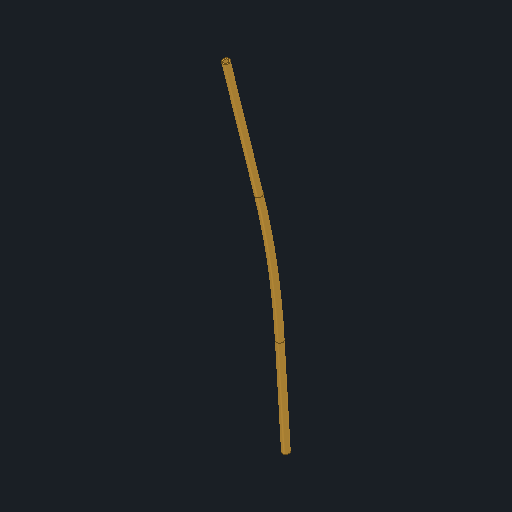
# Autodesk Inventor part: prop_shaft
Saved by Autodesk Inventor 2023 (Build 270158030, 158C)
## iProperties
Created: 2022-04-18
Part Number: prop_shaft
Material: Generic
Document SubType Name: Modeling
Designer: kardo
Density: 1 g/cm^3
Appearance: Brass - Prop shaft
Author: kardo
Autodesk Inventor part; units mm, degrees
ref_plane "YZ Plane" through (0, 0, 0) normal (1, 0, 0) x (0, 1, 0)
ref_plane "XZ Plane" through (0, 0, 0) normal (0, 1, 0) x (-1, 0, 0)
ref_plane "XY Plane" through (0, 0, 0) normal (0, 0, 1) x (1, 0, 0)
derived "stencil_frame.ipt"
sketch "sk_drivetrain_profile" plane through (6, 0, 0) normal (1, 0, 0) x (0, 1, 0)
  line L0 (-547.3485, 0) -> (393.091, 0) construction
  line L1 (-363, 4666.1952) -> (-363, -2045.0469) construction
  line L2 (0, 4666.1952) -> (0, -2045.0469) construction
  line L3 (-140.6277, 54.4571) -> (-133.8539, 27.2888)
  line L4 (-388, 0) -> (-343.0839, 2.7472)
  line L5 (-137.2408, 40.8729) -> (-226.9463, 18.5069)
  line L6 (-320.2745, 4.1423) -> (-272.9504, 7.0367) construction
  line L7 (-272.9504, 7.0367) -> (-226.9463, 18.5069) construction
  line L8 (-133.8539, 27.2888) -> (-133.8539, 22.2888) construction
  line L9 (-343.0839, 2.7472) -> (-320.2745, 4.1423)
  line L10 (-1246.9714, 4491.7596) -> (383.4376, -2047.4538) construction
  line L11 (-227.5223, 20.8174) -> (-137.8168, 43.1835) construction
  line L12 (-136.6647, 38.5624) -> (-226.3702, 16.1963) construction
  line L13 (-227.5223, 20.8174) -> (-226.3702, 16.1963) construction
  spline S0 degree 2 poles (-320.2745, 4.1423) (-272.9504, 7.0367) (-226.9463, 18.5069) knots 1 1 1 2 2 2
  line L14 (0, 21.4767) -> (-254.1001, 20.7404) construction
  line L15 (-55.6943, 22.5153) -> (-309.842, 21.7788) construction
  point P0 (0, 0)
  point P1 (-217.5636, 20.8462)
  point P2 (-207.6048, 20.8751)
  point P3 (-202.7352, 22.0892)
ref_plane "plane_motor_mount" through (0, -127.05, 0) normal (0, 0.9702957, 0.2419219) x (-1, 0, 0)
sketch "sk_prop_shaft_profile" plane through (0, -127.05, 0) normal (0, 0.9702957, 0.2419219) x (-1, 0, 0)
  circle A0 centre (-6, 42.1242) radius 2.3812
  point P0 (0, -30.7362)
  dimension "d1" = 4.7625
  constraints: 1 centre point, 1 coincident
  measures "d1" diameter of A0
derived "parameters_powertrain.ipt"
sweep "Sweep1" add profiles "sk_prop_shaft_profile" path "sk_drivetrain_profile" path curves L5 S0 L9 L4
shell "Shell1" thickness 0.7937 removed faces 2 at (6.4028, -388.0321, 0.5254) at (5.542, -137.2345, 40.8479)
equation "\"d1\" = prop_shaft_od"
equation "\"prop_shaft_od\" = 4.7625"
body "Solid1"
